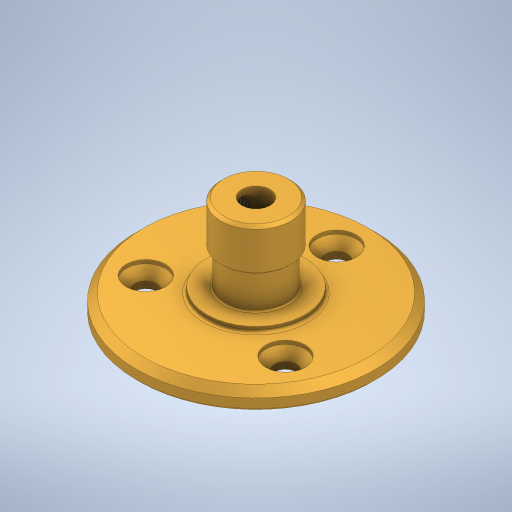
# Autodesk Inventor part: wheelHub
Saved by Autodesk Inventor 2023 (Build 270158000, 158)
## iProperties
Created: 2023-06-24
Part Number: wheelHub
Material: Латунь, мягкая, желтая
Document SubType Name: Modeling
Designer: khrip
Density: 8.47 g/cm^3
Appearance: Латунь — сатинированная
Author: khrip
Autodesk Inventor part; units mm, degrees
ref_plane "YZ Plane" through (0, 0, 0) normal (1, 0, 0) x (0, 1, 0)
ref_plane "XZ Plane" through (0, 0, 0) normal (0, 1, 0) x (-1, 0, 0)
ref_plane "XY Plane" through (0, 0, 0) normal (0, 0, 1) x (1, 0, 0)
sketch "Эскиз1" plane through (0, 0, 0) normal (1, 0, 0) x (0, 1, 0)
  line L0 (0, 0) -> (2.7, 0)
  line L1 (2.7, -7.4) -> (2.7, -17)
  line L2 (2.7, -17) -> (0, -17)
  line L3 (0, -17) -> (0, 0)
  line L4 (3.1, -7) -> (3.45, -7)
  line L5 (3.45, -7) -> (3.45, -4.4)
  line L6 (3.45, 0) -> (2.7, 0)
  arc A0 (3.1, -7) -> (2.7, -7.4) centre (3.1, -7.4) ccw
  line L7 (3.45, 0) -> (8.45, 0)
  line L8 (8.45, -4.4) -> (3.45, -4.4)
  line L9 (8.45, 0) -> (10.45, 0)
  line L10 (10.45, -5) -> (8.45, -5)
  line L11 (8.45, -5) -> (8.45, -4.4)
  line L12 (10.45, 0) -> (14.45, 0)
  line L13 (14.45, -2) -> (14.45, -5)
  line L14 (14.45, -5) -> (10.45, -5)
  line L15 (14.45, 0) -> (5.45, 0)
  line L16 (5.45, 0) -> (5.45, -2)
  line L17 (5.45, -2) -> (14.45, -2)
  point P0 (5.45, 0)
  dimension "d0" = 2.7
  dimension "d1" = 17
  dimension "d4" = 7
  dimension "d5" = 0.4
  dimension "d6" = 0.75
  dimension "d7" = 5
  dimension "d15" = 4
  dimension "d16" = 9
  dimension "d17" = 2
  constraints: 36 end point, 7 horizontal, 7 parallel, 4 perpendicular, 2 point on circle, 2 tangent, 1 centre point, 1 point on line
  measures "d0" distance of L1.end L2.end
  measures "d1" distance of L0.end L1.end
  measures "d4" distance between parallel lines of L6 L4
  measures "d5" radius of A0
  measures "d6" distance between parallel lines of L1 L5
  measures "d7" distance of L8.start L5.end
  measures "d15" distance of L13.end L14.end
  measures "d16" distance of L13.start L16.end
  measures "d17" distance between parallel lines of L7 L17
revolve "Вращение1" add sketch "Эскиз1" angle 360 about axis through (0, 0, 0) along (0, 1, 0)
fillet "Сопряжение1" radius 0.25 1 edges at (0, 3.45, 4.4)
fillet "Сопряжение2" radius 0.25 1 edges at (0, 8.45, 4.4)
chamfer "Фаска1" distance 0.25 angle 45 1 edges at (0, 8.45, 5)
chamfer "Фаска2" distance 0.4 angle 45 1 edges at (0, 14.45, 5)
chamfer "Фаска3" distance 1 angle 45 1 edges at (0, 2.7, 17)
sketch "Эскиз2" plane through (0, 0, 0) normal (0, -1, 0) x (1, 0, 0)
  circle A0 centre (0, 0) radius 2 projected
  circle A1 centre (0, 0) radius 3.1206
  constraints: 1 centre point, 1 coincident
hole "Отверстие1" at (0, 0, 0) direction (0, 1, 0) diameter 3.242 depth 11.8 tip angle 118 countersink diameter 4 countersink angle 90 thread size "M4x0.7" class "6H" standard "ISO Metric profile"
chamfer "Фаска4" distance 0.4 angle 45 1 edges at (0, 0, 17)
sketch "Эскиз3" plane through (0, 0, 0) normal (1, 0, 0) x (0, 1, 0)
  circle A0 centre (11.95, 0) radius 1.5
  line L0 (8.45, -4.75) -> (8.45, 4.75) projected
  point P0 (0, 0)
  dimension "d40" = 3
  dimension "d41" = 3.5
  constraints: 1 centre point
  measures "d40" diameter of A0
  measures "d41" distance from line of L0 A0.centre
hole "Отверстие2" at (0, 11.95, 0) direction (-1, 0, 0) diameter 2.459 depth 8.8 tip angle 118 countersink diameter 4 countersink angle 90 thread size "M3x0.5" class "6H" standard "ISO Metric profile"
chamfer "Фаска5" distance 0.4 angle 45 2 edges at (-1.5774, 11.9499, 1.2295) (-4.8465, 11.9473, 1.2295)
sketch "Эскиз4" plane through (0, 2.7, 0) normal (0, 1, 0) x (1, 0, 0)
  circle A0 centre (0, 0) radius 11.5
  circle A1 centre (0, 11.5) radius 2.8
  circle A2 centre (-9.9593, -5.75) radius 2.8
  circle A3 centre (9.9593, -5.75) radius 2.8
  dimension "d52" = 23
  dimension "d53" = 5.6
  dimension "d56" = 360
  constraints: 3 centre point, 1 coincident, 1 vertical alignment, 9 other
  measures "d53" diameter of A1
extrude "Выдавливание1" cut sketch "Эскиз4" against normal blind 0.5 contours A1 A0 | A0 A1 | A3 A0 | A0 A3 | A2 A0 | A0 A2
sketch "Эскиз5" plane through (-9.9593, 2.2, 5.75) normal (0, 1, 0) x (1, 0, 0)
  circle A0 centre (0, 0) radius 2.8 projected
  circle A1 centre (19.9186, 0) radius 2.8 projected
  circle A2 centre (9.9593, 17.25) radius 2.8 projected
  circle A3 centre (9.9593, 5.75) radius 1.621 projected
  circle A4 centre (9.9593, 5.75) radius 16.5 projected
hole "Отверстие3" at (-9.9593, 2.2, 5.75) at (9.9593, 2.2, 5.75) at (0, 2.2, -11.5) direction (0, -1, 0) diameter 3.1 depth 8.8 tip angle 118 countersink diameter 5.6 countersink angle 90 clearance for "Винт с потайной головкой ISO 2009/7046" size "M3" standard "ISO"
